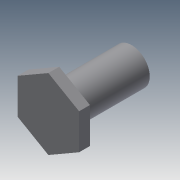
# Autodesk Inventor part: M10bolt
Saved by Autodesk Inventor 2015 (Build 190159000, 159)
## iProperties
Created: 2014-08-31
Part Number: M10bolt
Material: Generic
Document SubType Name: Modeling
Designer: shohei
Density: 1 g/cm^3
Appearance: Default
Author: shohei
Autodesk Inventor part; units mm, degrees
ref_plane "YZ Plane" through (0, 0, 0) normal (1, 0, 0) x (0, 1, 0)
ref_plane "XZ Plane" through (0, 0, 0) normal (0, 1, 0) x (-1, 0, 0)
ref_plane "XY Plane" through (0, 0, 0) normal (0, 0, 1) x (1, 0, 0)
sketch "Sketch1" plane through (0, 0, 0) normal (0, 1, 0) x (-1, 0, 0)
  line L0 (0, 9.8) -> (8.487, 4.9)
  line L1 (8.487, 4.9) -> (8.487, -4.9)
  line L2 (8.487, -4.9) -> (0, -9.8)
  line L3 (0, -9.8) -> (-8.487, -4.9)
  line L4 (-8.487, -4.9) -> (-8.487, 4.9)
  line L5 (-8.487, 4.9) -> (0, 9.8)
  point P0 (0, 0)
  point P1 (0, 0)
  dimension "d3" = 19.6
  constraints: 12 end point, 1 coincident, 13 other
  measures "d3" distance of L2.end L0.start
extrude "Extrusion1" add sketch "Sketch1" along normal blind 3
sketch "Sketch2" plane through (0, 3, 0) normal (0, 1, 0) x (1, 0, 0)
  circle A0 centre (0, 0) radius 5
  dimension "d4" = 10
  constraints: 1 centre point, 1 coincident
  measures "d4" diameter of A0
extrude "Extrusion2" add sketch "Sketch2" along normal blind 20
body "Solid1"
